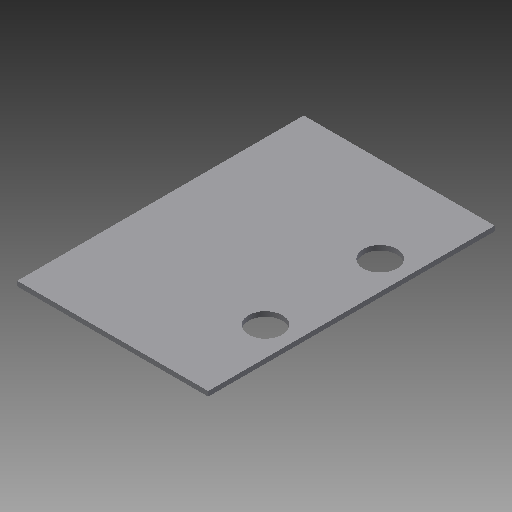
# Autodesk Inventor part: Shielding side
Saved by Autodesk Inventor 2018 (Build 220112000, 112)
## iProperties
Created: 2015-04-20
Part Number: Shielding side
Material: Generic
Document SubType Name: Modeling
Designer: Pascal
Density: 1 g/cm^3
Appearance: Default
Author: Pascal
Autodesk Inventor part; units mm, degrees
ref_plane "YZ Plane" through (0, 0, 0) normal (1, 0, 0) x (0, 1, 0)
ref_plane "XZ Plane" through (0, 0, 0) normal (0, 1, 0) x (-1, 0, 0)
ref_plane "XY Plane" through (0, 0, 0) normal (0, 0, 1) x (1, 0, 0)
sketch "Sketch1" plane through (0, 0, 0) normal (0, 1, 0) x (-1, 0, 0)
  line L0 (12.2137, 18.6426) -> (-13.1863, 18.6426)
  line L1 (-13.1863, 18.6426) -> (-13.1863, -19.4574)
  line L2 (-13.1863, -19.4574) -> (12.2137, -19.4574)
  line L3 (12.2137, -19.4574) -> (12.2137, 18.6426)
  point P0 (0, 0)
  dimension "d0" = 25.4
  dimension "d1" = 38.1
  constraints: 8 end point, 2 parallel, 1 horizontal, 1 perpendicular
  measures "d0" distance of L0.start L0.end
  measures "d1" distance of L2.end L0.start
extrude "Extrusion1" add sketch "Sketch1" along normal blind 0.635
hole "Hole1" at (9.3763, 0.635, 7.2126) direction (0, -1, 0) diameter 4.4958 depth 0.635 clearance for "Flat Head Machine Screw (82)" size "#8" standard "Ansi Unified Screw Threads"
hole "Hole5" at (9.3763, 0.635, -8.0274) direction (0, -1, 0) diameter 4.4958 depth 25.4 clearance for "Flat Head Machine Screw (82)" size "#8" standard "Ansi Unified Screw Threads"
body "Solid1"
